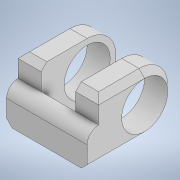
# Autodesk Inventor part: dhillg25_Lab2
Saved by Autodesk Inventor 2021 (Build 250183000, 183)
## iProperties
Created: 2020-09-23
Part Number: dhillg25_Lab2
Material: Generic
Document SubType Name: Modeling
Designer: gurle
Mass: 84.003 g
Surface Area: 225.175 cm^2
Volume: 84.003 cm^3
Density: 1 g/cm^3
Appearance: Default
Author: gurle
Autodesk Inventor part; units mm, degrees
ref_plane "YZ Plane" through (0, 0, 0) normal (1, 0, 0) x (0, 1, 0)
ref_plane "XZ Plane" through (0, 0, 0) normal (0, 1, 0) x (-1, 0, 0)
ref_plane "XY Plane" through (0, 0, 0) normal (0, 0, 1) x (1, 0, 0)
sketch "Sketch1" plane through (0, 0, 0) normal (0, 1, 0) x (-1, 0, 0)
  line L0 (0, 0) -> (70, 0)
  line L1 (70, 0) -> (70, -84.6705) construction
  line L2 (0, -84.6705) -> (0, 0) construction
  line L3 (70, 0) -> (0, 0) construction
  line L4 (0, 0) -> (0, -75)
  line L5 (0, -75) -> (20, -75)
  line L6 (20, -75) -> (20, -10)
  line L7 (20, -10) -> (50, -10)
  line L8 (50, -10) -> (50, -75)
  line L9 (50, -75) -> (70, -75)
  line L10 (70, -75) -> (70, 0)
  dimension "d0" = 70
  dimension "d1" = 20
  dimension "d2" = 30
  dimension "d3" = 20
  dimension "d4" = 10
  dimension "d20" = 65
  constraints: 22 end point, 5 perpendicular, 2 horizontal, 2 point on line, 1 parallel, 1 vertical
  measures "d0" distance of L0.start L0.end
  measures "d1" distance of L4.end L5.end
  measures "d2" distance of L6.end L7.end
  measures "d3" distance of L8.end L9.end
  measures "d4" distance between parallel lines of L0 L7
  measures "d20" distance of L5.end L6.end
extrude "Extrusion1" add sketch "Sketch1" along normal blind 50
sketch "Sketch2" plane through (0, 50, 0) normal (0, 1, 0) x (1, 0, 0)
  line L0 (-70, 0) -> (0, 0) projected
  line L1 (0, 0) -> (-70, 0)
  line L2 (-70, 0) -> (-70, 10)
  line L3 (-70, 10) -> (0, 10)
  line L4 (0, 10) -> (0, 0)
  dimension "d7" = 70
  dimension "d8" = 10
  constraints: 8 end point, 2 parallel, 1 horizontal, 1 perpendicular
  measures "d7" distance of L2.end L3.end
  measures "d8" distance of L1.end L2.end
extrude "Extrusion2" cut sketch "Sketch2" against normal blind 20
fillet "Fillet1" radius 10 1 edges at (-35, 30, 0)
fillet "Fillet2" radius 25 4 edges at (-10, 50, -75) (-10, 0, -75) (-60, 0, -75) (-60, 50, -75)
chamfer "Chamfer1" distance 5 angle 45 8 edges at (0, 0, -25.0003) (0, 42.6778, -67.6778) (0, 50, -30.0003) (-70, 50, -30.0002) (-70, 7.3222, -67.6778) (-70, 0, -25.0002) (-60, 50, -10) (-10, 50, -10)
sketch "Sketch4" plane through (0, 25, -50) normal (1, 0, 0) x (0, 0, -1)
  circle A0 centre (0, 0) radius 20
  point P0 (-50, -25)
  dimension "d17" = 40
  constraints: 1 centre point
  measures "d17" diameter of A0
extrude "Extrusion3" cut sketch "Sketch4" against normal through all
body "Solid1"
